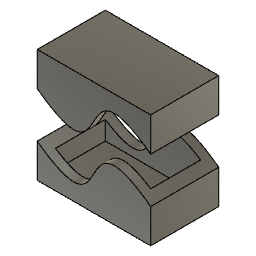
hollowbox (Autodesk Fusion 360 design; units mm, degrees)
Autodesk Fusion 360 part; units mm, degrees
note: some values were not read from the file. Chosen so that the rebuilt part matches the saved one: which bodies a step acts on.
sketch "Sketch1" plane through (0, 0, 0) normal (0, 0, 1) x (1, 0, 0)
  line L0 (0, 0) -> (50, 0)
  line L1 (50, 0) -> (50, 30)
  line L2 (50, 30) -> (0, 30)
  line L3 (0, 30) -> (0, 0)
  dimension "d1" = 30
  dimension "d2" = 50
  constraint horizontal L0
  constraint vertical L1
  constraint horizontal L2
  constraint vertical L3
  constraint coincident L0.start L3.end
  measures "d1" distance of L0.start L2.end
  measures "d2" distance of L0.start L0.end
extrude "Extrude1" add sketch "Sketch1" along normal blind 30 makes body 1
shell "Shell1" thickness 4 removed faces 0 bodies 1
sketch "Sketch2" plane through (0, 0, 0) normal (0, -1, 0) x (1, 0, 0)
  line L0 (0, 0) -> (50, 0)
  line L1 (50, 0) -> (50, 30)
  line L2 (50, 30) -> (0, 30)
  line L3 (0, 30) -> (0, 0)
  spline S0 degree 5 poles (0, 15) (0.8973, 14.3396) (2.6486, 13.0903) (5.1454, 11.4312) (8.2134, 9.6502) (11.6094, 8.1486) (14.5671, 7.3716) (17.096, 7.3044) (19.2202, 7.9088) (20.9851, 9.1129) (22.4631, 10.8009) (23.745, 12.8266) (24.9327, 15.0237) (26.132, 17.2168) (27.4453, 19.2314) (28.9669, 20.904) (30.7785, 22.0916) (32.9432, 22.6818) (35.5003, 22.6046) (38.4701, 21.8233) (41.8603, 20.3238) (44.9083, 18.5499) (47.3816, 16.899) (49.1134, 15.6566) (50, 15) knots 0 0 0 0 0 0 0.05 0.1 0.15 0.2 0.25 0.3 0.35 0.4 0.45 0.5 0.55 0.6 0.65 0.7 0.75 0.8 0.85 0.9 0.95 1 1 1 1 1 1
  point P0 (19, 8)
  point P1 (24.923, 15)
  point P2 (31, 22)
  constraint midpoint L3 S0.start
  constraint midpoint L1 S0.end
split "Split1" by curves path "Sketch2" along S0 bodies 1 makes body 2 at (16.6667, 20, 0)
move_body "Move1" bodies 1 to x (1, 0, 0) y (0, 1, 0) z (0, 0, 1) at (0, 0, 20)
